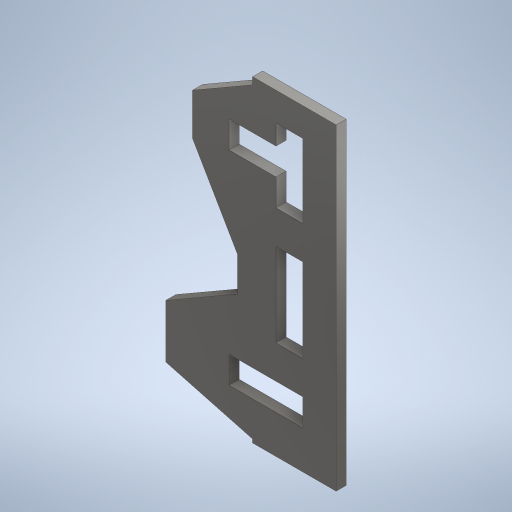
# Autodesk Inventor part: act_p1_KUMAR
Saved by Autodesk Inventor 2024 (Build 280153000, 153)
## iProperties
Created: 2024-10-02
Part Number: act_p1_KUMAR
Material: Steel, Mild
Document SubType Name: Modeling
Designer: NK
Density: 7.85 g/cm^3
Appearance: Semi-Polished
Mass: 571.675 g
Surface Area: 302.794 cm^2
Volume: 72.8249 cm^3
Author: NK
Autodesk Inventor part; units mm, degrees
ref_plane "YZ Plane" through (0, 0, 0) normal (1, 0, 0) x (0, 1, 0)
ref_plane "XZ Plane" through (0, 0, 0) normal (0, 1, 0) x (-1, 0, 0)
ref_plane "XY Plane" through (0, 0, 0) normal (0, 0, 1) x (1, 0, 0)
sketch "Sketch1" plane through (0, 0, 0) normal (0, 1, 0) x (-1, 0, 0)
  line L0 (14.7222, -35.3265) -> (64.7222, -35.3265)
  line L1 (64.7222, -35.3265) -> (64.7222, -39.5419)
  line L2 (64.7222, -39.5419) -> (100.7222, -60.3265)
  line L3 (100.7222, -60.3265) -> (100.7222, -85.3265)
  line L4 (100.7222, -85.3265) -> (73.7222, -132.0919)
  line L5 (73.7222, -132.0919) -> (73.7222, -152.5004)
  line L6 (73.7222, -152.5004) -> (116.7222, -177.3265)
  line L7 (116.7222, -209.3265) -> (64.7222, -223.2598)
  line L8 (64.7222, -223.2598) -> (64.7222, -225.3265)
  line L9 (64.7222, -225.3265) -> (14.7222, -225.3265)
  line L10 (78.7222, -64.3265) -> (50.7222, -64.3265)
  line L11 (50.7222, -64.3265) -> (50.7222, -52.3265)
  line L12 (50.7222, -52.3265) -> (34.7222, -52.3265)
  line L13 (34.7222, -52.3265) -> (34.7222, -96.3265)
  line L14 (34.7222, -96.3265) -> (50.7222, -96.3265)
  line L15 (50.7222, -96.3265) -> (50.7222, -80.3265)
  line L16 (50.7222, -80.3265) -> (78.7222, -80.3265)
  line L17 (78.7222, -80.3265) -> (78.7222, -64.3265)
  line L18 (50.7222, -116.3265) -> (34.7222, -116.3265)
  line L19 (34.7222, -116.3265) -> (34.7222, -166.3265)
  line L20 (34.7222, -166.3265) -> (50.7222, -166.3265)
  line L21 (50.7222, -166.3265) -> (50.7222, -116.3265)
  line L22 (78.7222, -186.3265) -> (34.7222, -186.3265)
  line L23 (34.7222, -186.3265) -> (34.7222, -202.3265)
  line L24 (34.7222, -202.3265) -> (78.7222, -202.3265)
  line L25 (78.7222, -202.3265) -> (78.7222, -186.3265)
  line L26 (116.7222, -177.3265) -> (116.7222, -209.3265)
  line L27 (14.7222, -35.3265) -> (14.7222, -225.3265)
  point P0 (0, 0)
  dimension "d2" = 25
  dimension "d3" = 25
  dimension "d4" = 92
  dimension "d5" = 32
  dimension "d6" = 16
  dimension "d10" = 35.3265
  dimension "d13" = 15
  dimension "d14" = 150
  dimension "d15" = 120
  dimension "d16" = 16
  dimension "d17" = 12
  dimension "d18" = 28
  dimension "d19" = 17
  dimension "d20" = 44
  dimension "d21" = 20
  dimension "d22" = 50
  dimension "d24" = 16
  dimension "d25" = 20
  dimension "d26" = 16
  dimension "d27" = 44
  dimension "d36" = 43
  dimension "d37" = 120
  dimension "d38" = 86
  dimension "d39" = 50
  dimension "d40" = 14.7222
  dimension "d41" = 102
  dimension "d42" = 50
  dimension "d43" = 20
  constraints: 56 end point, 13 vertical, 9 horizontal, 3 point on line, 1 collinear, 1 parallel, 1 perpendicular
  measures "d2" distance from line of L2.end L0
  measures "d3" distance of L3.end L2.end
  measures "d4" vertical distance of L6.end L3.end
  measures "d5" distance of L7.start L6.end
  measures "d6" distance from line of L9 L7.start
  measures "d10" distance from line of point (0, 0) L0
  measures "d13" angle of L9 L7
  measures "d14" angle of L3 L4
  measures "d15" angle of L3 L2
  measures "d16" distance between parallel lines of L16 L10
  measures "d17" distance between parallel lines of L12 L10
  measures "d18" distance between parallel lines of L15 L17
  measures "d19" distance between parallel lines of L12 L0
  measures "d20" distance between parallel lines of L14 L12
  measures "d21" distance between parallel lines of L18 L14
  measures "d22" distance between parallel lines of L20 L18
  measures "d24" distance between parallel lines of L19 L21
  measures "d25" distance between parallel lines of L20 L22
  measures "d26" distance between parallel lines of L24 L22
  measures "d27" distance between parallel lines of L23 L25
  measures "d36" distance between parallel lines of L5 L26
  measures "d37" angle of L26 L6
  measures "d38" distance between parallel lines of L27 L3
  measures "d39" distance between parallel lines of L27 L1
  measures "d40" distance from line of point (0, 0) L27
  measures "d41" distance between parallel lines of L26 L27
  measures "d42" distance between parallel lines of L27 L8
  measures "d43" distance between parallel lines of L19 L27
extrude "Extrusion1" add sketch "Sketch1" along normal blind 6
body "Solid1"
